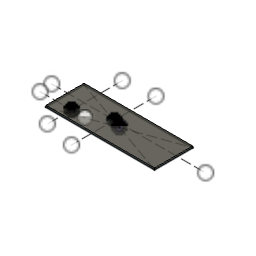
cover_back v3 (Autodesk Fusion 360 design; units mm, degrees)
Autodesk Fusion 360 part; units mm, degrees
sketch "Skizze1" plane through (0, 0, 0) normal (0, 0, 1) x (1, 0, 0)
  line L0 (74, -26) -> (-74, -26)
  line L1 (-74, -26) -> (-74, 26)
  line L2 (-74, 26) -> (74, 26)
  line L3 (74, 26) -> (74, -26)
  line L4 (74, -26) -> (-74, 26) construction
  line L5 (-74, -26) -> (74, 26) construction
  line L6 (-11.75, 61.7133) -> (-11.75, -53.3839) construction
  line L7 (-97.1763, 5.1) -> (112.5731, 5.1) construction
  line L8 (-53, 57.008) -> (-53, -45) construction
  line L9 (-95.9922, -11.9) -> (-35, -11.9) construction
  circle A0 centre (-53, -11.9) radius 4.5
  line L10 (-6.25, 0.35) -> (-17.25, 0.35)
  line L11 (-17.25, 0.35) -> (-17.25, 9.85)
  line L12 (-17.25, 9.85) -> (-6.25, 9.85)
  line L13 (-6.25, 9.85) -> (-6.25, 0.35)
  line L14 (-6.25, 0.35) -> (-17.25, 9.85) construction
  line L15 (-17.25, 0.35) -> (-6.25, 9.85) construction
  point P0 (-53, -11.9)
  point P1 (-11.75, 5.1)
  dimension "d1" = 148
  dimension "d2" = 52
  dimension "d3" = 62.25
  dimension "d4" = 20.9
  dimension "d6" = 21
  dimension "d8" = 37.9
  dimension "d9" = 9
  dimension "d12" = 11
  dimension "d13" = 9.5
  constraint horizontal L0
  constraint perpendicular L0 L1
  constraint parallel L0 L2
  constraint parallel L1 L3
  constraint coincident L4 origin
  constraint coincident L5 origin
  constraint perpendicular L2 L6
  constraint horizontal L7
  constraint perpendicular L2 L8
  constraint horizontal L9
  constraint coincident L8 P0
  constraint coincident L9 P0
  constraint coincident P0 A0.centre
  constraint horizontal L10
  constraint perpendicular L10 L11
  constraint parallel L10 L12
  constraint parallel L11 L13
  constraint coincident L14 P1
  constraint coincident L15 P1
  constraint coincident L7 P1
  constraint coincident L6 P1
  measures "d1" distance of L1 L3
  measures "d2" distance of L0 L2
  measures "d3" distance of L1 L6
  measures "d4" distance of L2 L7
  measures "d6" distance of L1 L8
  measures "d8" distance of L2 L9
  measures "d9" diameter of A0
  measures "d12" distance of L11 L13
  measures "d13" distance of L10 L12
extrude "Extrusion1" add sketch "Skizze1" along normal blind 2
